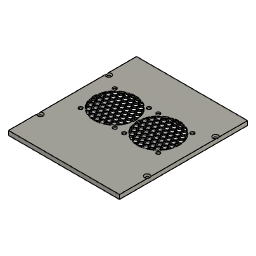
Top v8 (Autodesk Fusion 360 design; units mm, degrees)
Autodesk Fusion 360 part; units mm, degrees
sketch "Sketch2" plane through (0, 0, 0) normal (0, 0, 1) x (1, 0, 0)
  line L0 (0, 0) -> (130, 0)
  line L1 (130, 0) -> (130, 150)
  line L2 (130, 150) -> (0, 150)
  line L3 (0, 150) -> (0, 0)
  dimension "d5" = 130
  dimension "d6" = 150
  constraint horizontal L0
  constraint vertical L1
  constraint horizontal L2
  constraint vertical L3
  constraint coincident L0.start L3.end
  measures "d5" distance of L0.start L0.end
  measures "d6" distance of L0.start L2.end
extrude "Extrude2" add sketch "Sketch2" along normal blind 5 makes body 1
sketch "Sketch3" plane through (0, 0, 5) normal (0, 0, 1) x (-1, 0, 0)
  line L0 (0, -150) -> (0, 0)
  line L1 (0, 0) -> (-130, 0)
  line L2 (-130, 0) -> (-130, -150)
  line L3 (-130, -150) -> (0, -150)
  line L4 (-5, -150) -> (-5, 0) construction
  line L5 (-125, -150) -> (-125, 0) construction
  point P0 (-2.5, -115)
  point P1 (-2.5, -35)
  point P2 (-127.5, -115)
  point P3 (-127.5, -35)
  dimension "d9" = 5
  dimension "d10" = 5
  dimension "d11" = 2.5
  dimension "d12" = 35
  dimension "d13" = 35
  dimension "d14" = 35
  dimension "d15" = 2.5
  dimension "d16" = 2.5
  dimension "d17" = 35
  constraint coincident L3 L4.start
  constraint coincident L1 L4.end
  constraint perpendicular L1 L4
  constraint coincident L3 L5.start
  constraint coincident L1 L5.end
  constraint perpendicular L1 L5
  measures "d9" distance of L0 L4
  measures "d10" distance of L2 L5
  measures "d11" distance of L0 P0
  measures "d12" distance of L3 P0
  measures "d13" distance of L1 P1
  measures "d14" distance of L3 P2
  measures "d15" distance of L2 P2
  measures "d16" distance of L2 P3
  measures "d17" distance of L1 P3
hole "Hole1" at (2.5, 115, 5) at (127.5, 115, 5) at (127.5, 35, 5) at (2.5, 35, 5) direction (0, 0, -1) diameter 3.4 depth 50 tip angle 180 countersink diameter 6.3 countersink angle 90 bodies 1
sketch "Sketch4" plane through (0, 0, 0) normal (0, 0, -1) x (1, 0, 0)
  circle A0 centre (127.5, -35) radius 1.7
  circle A1 centre (2.5, -115) radius 1.7
  circle A2 centre (127.5, -115) radius 1.7
  circle A3 centre (2.5, -35) radius 1.7
  line L0 (0, 0) -> (0, -150)
  line L1 (0, -150) -> (130, -150)
  line L2 (130, -150) -> (130, 0)
  line L3 (130, 0) -> (0, 0)
  line L4 (5, 0) -> (5, -150) construction
  line L5 (125, 0) -> (125, -150) construction
  line L6 (0, -40) -> (130, -40) construction
  line L7 (14, -59.5) -> (116, -59.5)
  line L8 (116, -59.5) -> (116, -110.5)
  line L9 (116, -110.5) -> (14, -110.5)
  line L10 (14, -110.5) -> (14, -59.5)
  line L11 (14, -85) -> (116, -85) construction
  dimension "d23" = 5
  dimension "d24" = 5
  dimension "d25" = 40
  dimension "d27" = 102
  dimension "d28" = 51
  dimension "d29" = 9
  dimension "d30" = 85
  constraint coincident L1 L4.end
  constraint perpendicular L1 L4
  constraint coincident L3 L5.start
  constraint coincident L1 L5.end
  constraint perpendicular L1 L5
  constraint coincident L0 L6.start
  constraint coincident L2 L6.end
  constraint perpendicular L2 L6
  constraint horizontal L7
  constraint vertical L8
  constraint horizontal L9
  constraint vertical L10
  constraint midpoint L10 L11.start
  constraint midpoint L8 L11.end
  measures "d23" distance of L0 L4
  measures "d24" distance of L2 L5
  measures "d25" distance of L3 L6
  measures "d27" distance of L7.start L7.end
  measures "d28" distance of L7.start L9.end
  measures "d29" distance of L5 L8
  measures "d30" distance of L3 L11
extrude "Extrude3" cut sketch "Sketch4" against normal blind 3.5 contours L7 L8 L9 L10 bodies 1
sketch "Sketch5" plane through (0, 0, 3.5) normal (0, 0, -1) x (1, 0, 0)
  line L0 (14, -110.5) -> (116, -110.5)
  line L1 (116, -110.5) -> (116, -59.5)
  line L2 (116, -59.5) -> (14, -59.5)
  line L3 (14, -59.5) -> (14, -110.5)
  line L4 (14.5, -60) -> (64.5, -60) construction
  line L5 (64.5, -60) -> (64.5, -110) construction
  line L6 (64.5, -110) -> (14.5, -110) construction
  line L7 (14.5, -110) -> (14.5, -60) construction
  line L8 (59.5, -105) -> (19.5, -105) construction
  line L9 (19.5, -105) -> (19.5, -65) construction
  line L10 (19.5, -65) -> (59.5, -65) construction
  line L11 (59.5, -65) -> (59.5, -105) construction
  line L12 (65, -59.5) -> (65, -110.5) construction
  line L13 (14, -85) -> (65, -85) construction
  line L14 (39.5, -60) -> (39.5, -110) construction
  circle A0 centre (39.5, -85) radius 25
  circle A1 centre (90.5, -85) radius 25
  point P0 (19.5, -65)
  point P1 (59.5, -65)
  point P2 (59.5, -105)
  point P3 (19.5, -105)
  point P4 (110.5, -65)
  point P5 (70.5, -65)
  point P6 (70.5, -105)
  point P7 (110.5, -105)
  dimension "d33" = 50
  dimension "d34" = 50
  dimension "d35" = 0.5
  dimension "d36" = 0.5
  dimension "d37" = 5
  constraint horizontal L4
  constraint vertical L5
  constraint horizontal L6
  constraint vertical L7
  constraint midpoint L2 L12.start
  constraint midpoint L0 L12.end
  constraint coincident P0 L9.end
  constraint coincident P1 L10.end
  constraint coincident P2 L8.start
  constraint coincident P3 L8.end
  constraint symmetric L12 P0 P4
  constraint symmetric L12 P1 P5
  constraint symmetric L12 P2 P6
  constraint symmetric L12 P3 P7
  constraint midpoint L3 L13.start
  constraint midpoint L12 L13.end
  constraint midpoint L4 L14.start
  constraint midpoint L6 L14.end
  constraint midpoint L14 A0.centre
  constraint coincident L14.start A0
  constraint symmetric L12 A0 A1
  measures "d33" distance of L4.start L4.end
  measures "d34" distance of L4.start L6.end
  measures "d35" distance of L2 L4
  measures "d36" distance of L3 L7
hole "Hole2" at (59.5, 65, 3.5) at (19.5, 65, 3.5) at (19.5, 105, 3.5) at (59.5, 105, 3.5) at (70.5, 105, 3.5) at (70.5, 65, 3.5) at (110.5, 65, 3.5) at (110.5, 105, 3.5) direction (0, 0, 1) diameter 4.4 depth 50 tip angle 180 bodies 1
sketch "Sketch6" plane through (0, 0, 3.5) normal (0, 0, -1) x (1, 0, 0)
  circle A0 centre (110.5, -65) radius 2.2
  circle A1 centre (70.5, -105) radius 2.2
  circle A2 centre (19.5, -105) radius 2.2
  circle A3 centre (59.5, -65) radius 2.2
  circle A4 centre (19.5, -65) radius 2.2
  circle A5 centre (59.5, -105) radius 2.2
  circle A6 centre (70.5, -65) radius 2.2
  circle A7 centre (110.5, -105) radius 2.2
  line L0 (14, -110.5) -> (116, -110.5)
  line L1 (116, -110.5) -> (116, -59.5)
  line L2 (116, -59.5) -> (14, -59.5)
  line L3 (14, -59.5) -> (14, -110.5)
  line L4 (65, -59.5) -> (65, -110.5) construction
  line L5 (14.5, -60) -> (64.5, -60) construction
  line L6 (64.5, -60) -> (64.5, -110) construction
  line L7 (64.5, -110) -> (14.5, -110) construction
  line L8 (14.5, -110) -> (14.5, -60) construction
  line L9 (39.5, -60) -> (39.5, -110) construction
  line L10 (14.5, -85) -> (64.5, -85) construction
  circle A8 centre (39.5, -85) radius 24.5
  line L11 (39.5, -88.4641) -> (42.5, -86.7321)
  line L12 (42.5, -86.7321) -> (42.5, -83.2679)
  line L13 (42.5, -83.2679) -> (39.5, -81.5359)
  line L14 (39.5, -81.5359) -> (36.5, -83.2679)
  line L15 (36.5, -83.2679) -> (36.5, -86.7321)
  line L16 (36.5, -86.7321) -> (39.5, -88.4641)
  line L17 (42.5, -86.7321) -> (45.5, -88.4641)
  line L18 (45.5, -88.4641) -> (48.5, -86.7321)
  line L19 (48.5, -86.7321) -> (48.5, -83.2679)
  line L20 (48.5, -83.2679) -> (45.5, -81.5359)
  line L21 (45.5, -81.5359) -> (42.5, -83.2679)
  line L22 (42.5, -83.2679) -> (42.5, -86.7321)
  line L23 (39.5, -85) -> (42.5, -85) construction
  line L24 (39.5, -85) -> (41, -82.4019) construction
  circle A9 centre (90.5, -85) radius 24.5
  line L25 (90.5, -81.5359) -> (93.5, -83.2679)
  line L26 (93.5, -83.2679) -> (93.5, -86.7321)
  line L27 (93.5, -86.7321) -> (90.5, -88.4641)
  line L28 (90.5, -88.4641) -> (87.5, -86.7321)
  line L29 (90.5, -85) -> (87.5, -85) construction
  line L30 (90.5, -85) -> (89, -82.4019) construction
  line L31 (87.5, -83.2679) -> (90.5, -81.5359)
  line L32 (84.5, -81.5359) -> (87.5, -83.2679)
  line L33 (87.5, -83.2679) -> (87.5, -86.7321)
  line L34 (87.5, -86.7321) -> (84.5, -88.4641)
  line L35 (84.5, -88.4641) -> (81.5, -86.7321)
  line L36 (81.5, -86.7321) -> (81.5, -83.2679)
  line L37 (81.5, -83.2679) -> (84.5, -81.5359)
  point P0 (39.5, -85)
  point P1 (45.5, -85)
  dimension "d41" = 50
  dimension "d42" = 50
  dimension "d43" = 0.5
  dimension "d44" = 0.5
  dimension "d49" = 49
  dimension "d54" = 6
  constraint midpoint L2 L4.start
  constraint midpoint L0 L4.end
  constraint horizontal L5
  constraint vertical L6
  constraint horizontal L7
  constraint vertical L8
  constraint midpoint L5 L9.start
  constraint midpoint L7 L9.end
  constraint midpoint L8 L10.start
  constraint midpoint L6 L10.end
  constraint midpoint L9 P0
  constraint coincident P0 A8.centre
  constraint vertical L15
  constraint coincident L12.end L13.start
  constraint coincident L11.end L12.start
  constraint midpoint L12 L23.end
  constraint midpoint L13 L24.end
  constraint symmetric L4 A8 A9
  constraint symmetric L4 L11.start L27.end
  constraint symmetric L4 L11.end L28.end
  constraint symmetric L4 L12.end L31.start
  constraint symmetric L4 L13.end L25.start
  constraint symmetric L4 L14.end L25.end
  constraint symmetric L4 L15.end L26.end
  constraint symmetric L4 L17.end L34.end
  constraint symmetric L4 L18.end L35.end
  constraint symmetric L4 L19.end L36.end
  constraint symmetric L4 L20.end L32.start
  constraint symmetric L4 P0 A9.centre
  constraint symmetric L4 L23.end L29.end
  constraint symmetric L4 L24.end L30.end
  measures "d41" distance of L5.start L5.end
  measures "d42" distance of L5.start L7.end
  measures "d43" distance of L2 L5
  measures "d44" distance of L3 L8
  measures "d49" diameter of A8
  measures "d54" distance of L12 L15
extrude "Extrude5" cut sketch "Sketch5" against normal blind 5 contours A0 | A1 bodies 1
extrude "Extrude6" add sketch "Sketch6" against normal up to surface (1.5 mm away) thin wall 0.5 inside separate body contours L12 L17 L18 L19 L20 L21 L22 makes body 2
extrude "Extrude7" add sketch "Sketch6" against normal up to surface (1.5 mm away) thin wall 0.5 inside contours L11 L12 L13 L14 L15 L16 L22 bodies 2
pattern_linear "R-Pattern1" count 11 spacing 6 along (1, 0, 0) both ways count 11 spacing 6 along (0.5, -0.866025, 0) both ways of "Extrude7"
extrude "Extrude8" cut sketch "Sketch6" against normal up to surface (1.5 mm away) contours A8 | L11 L12 L13 L14 L15 L16 L22 | L12 L17 L18 L19 L20 L21 L22 keep common part bodies 2
extrude "Extrude9" add sketch "Sketch6" against normal up to surface (1.5 mm away) thin wall 1 outside contours A8 | L11 L12 L13 L14 L15 L16 L22 | L12 L17 L18 L19 L20 L21 L22 bodies 1 2
extrude "Extrude10" add sketch "Sketch6" against normal up to surface (1.5 mm away) thin wall 0.5 inside separate body contours L32 L33 L34 L35 L36 L37 makes body 3
extrude "Extrude11" add sketch "Sketch6" against normal up to surface (1.5 mm away) thin wall 0.5 inside contours L25 L26 L27 L28 L31 L33 bodies 3
pattern_linear "R-Pattern2" count 11 spacing 6 along (-1, 0, 0) both ways count 11 spacing 6 along (-0.5, -0.866025, 0) both ways of "Extrude11"
extrude "Extrude12" cut sketch "Sketch6" against normal up to surface (1.5 mm away) contours A9 | L25 L26 L27 L28 L31 L33 | L32 L33 L34 L35 L36 L37 keep common part bodies 3
extrude "Extrude13" add sketch "Sketch6" against normal up to surface (1.5 mm away) thin wall 1 outside contours A9 | L25 L26 L27 L28 L31 L33 | L32 L33 L34 L35 L36 L37 bodies 1 3
equation "d27 = ( 51 * 2 ) * 1 mm"
equation "Walls = 1 mm"
equation "Hexagon = 6 mm"
equation "OD = 51 mm"
equation "d49 = OD - Walls * 2"
equation "d54 = Hexagon"
equation "d55 = Walls / 2"
equation "d58 = Walls / 2"
equation "d63 = Hexagon"
equation "d64 = Hexagon"
equation "d67 = Walls"
equation "d70 = Walls / 2"
equation "d73 = Walls / 2"
equation "d78 = Hexagon"
equation "d79 = Hexagon"
equation "d82 = Walls"
